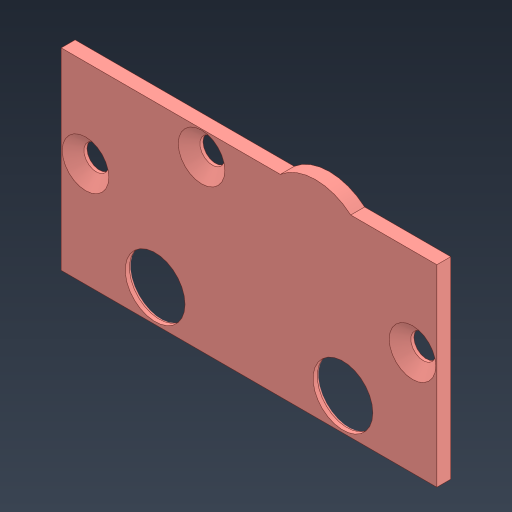
# Autodesk Inventor part: gearbox-wall-left
Saved by Autodesk Inventor 2023 (Build 270158000, 158)
## iProperties
Created: 2025-04-19
Part Number: gearbox-wall-left
Material: Generic
Document SubType Name: Modeling
Designer: szymo
Density: 1 g/cm^3
Appearance: Default(1)
Mass: 2.53528 g
Surface Area: 31.5747 cm^2
Volume: 2.53528 cm^3
Author: szymo
Autodesk Inventor part; units mm, degrees
ref_plane "YZ Plane" through (0, 0, 0) normal (1, 0, 0) x (0, 1, 0)
ref_plane "XZ Plane" through (0, 0, 0) normal (0, 1, 0) x (-1, 0, 0)
ref_plane "XY Plane" through (0, 0, 0) normal (0, 0, 1) x (1, 0, 0)
sketch "Sketch1" plane through (0, 0, 0) normal (0, 0, 1) x (1, 0, 0)
  circle A0 centre (-23.5, 0.7602) radius 2.5 projected
  circle A1 centre (23.5, 0.7602) radius 2.5 projected
  circle A2 centre (-6.8229, 9.9421) radius 2.5 projected
  arc A3 (-6.2914, -1.4253) -> (-23.3552, -14.2579) centre (-13.5, -9.6013) ccw projected
  arc A4 (-4.408, 0.1593) -> (-6.2914, -1.4253) centre (0, -6.9912) ccw projected
  arc A5 (23.3552, -14.2579) -> (18.5289, 0.0693) centre (13.5, -9.6013) ccw projected
  line L0 (-27, -14.2579) -> (27, -14.2579)
  circle A6 centre (-13.5, -9.6013) radius 6 projected
  circle A7 centre (13.5, -9.6013) radius 6 projected
  circle A8 centre (-13.5, -9.6013) radius 6.3
  circle A9 centre (13.5, -9.6013) radius 6.3
  arc A10 (15.8884, 4.2462) -> (2.7919, 9.881) centre (9.5585, 7.571) ccw projected
  arc A11 (18.5289, 0.0693) -> (15.8884, 4.2462) centre (13.15, -0.4079) ccw projected
  line L1 (23.3552, -14.2579) -> (27, -14.2579) projected
  line L2 (27, -14.2579) -> (27, 13.4421) projected
  line L3 (27, 13.4421) -> (14.6174, 13.4421) projected
  arc A12 (14.6174, 13.4421) -> (4.4995, 13.4421) centre (9.5585, 7.571) ccw projected
  line L4 (4.4995, 13.4421) -> (-27, 13.4421) projected
  line L5 (-27, 13.4421) -> (-27, -14.2579) projected
  line L6 (-27, -14.2579) -> (-23.3552, -14.2579) projected
  arc A13 (2.7919, 9.881) -> (-4.408, 0.1593) centre (2.2557, 2.7511) ccw projected
  point P0 (0, 0)
  point P1 (4.2365, 13.4421)
  point P2 (-17.7433, -14.2579)
  point P3 (-9.2567, -14.2579)
  point P4 (9.2567, -14.2579)
  point P5 (17.7433, -14.2579)
  point P6 (-23.3552, -14.2579)
  point P7 (23.3552, -14.2579)
  dimension "d0" = 0.3
  dimension "d1" = 0.3
  constraints: 2 centre point, 2 end point
  measures "d0" radial gap between concentric circles of A6 A8
  measures "d1" radial gap between concentric circles of A7 A9
ref_plane "Work Plane1" through (-19.5, -15.6013, 1) normal (0, 0, 1) x (1, 0, 0)
extrude "Extrusion1" add sketch "Sketch1" along normal up to surface (1 mm away) contours A0 | A1 | A2 | A4 A13 A10 A11 A5 L0 A9 A8 A3 | A3 L0 L5 L4 A12 L3 L2 A5 A11 A10 A13 A4
sketch "Sketch2" plane through (-27, 13.4421, 1) normal (0, 0, 1) x (1, 0, 0)
  line L0 (36.2567, -27.7) -> (17.7433, -27.7) projected
  circle A0 centre (13.5, -23.0433) radius 4 projected
  circle A1 centre (40.5, -23.0433) radius 4 projected
  arc A2 (17.7433, -27.7) -> (9.2567, -27.7) centre (13.5, -23.0433) ccw projected
  line L1 (9.2567, -27.7) -> (17.7433, -27.7)
  line L2 (36.2567, -27.7) -> (44.7433, -27.7)
  arc A3 (44.7433, -27.7) -> (36.2567, -27.7) centre (40.5, -23.0433) ccw projected
  circle A4 centre (13.5, -23.0433) radius 4.3
  circle A5 centre (40.5, -23.0433) radius 4.3
  line L3 (9.2567, -27.7) -> (0, -27.7) projected
  arc A6 (17.7433, -27.7) -> (9.2567, -27.7) centre (13.5, -23.0433) ccw projected
  arc A7 (44.7433, -27.7) -> (36.2567, -27.7) centre (40.5, -23.0433) ccw projected
  line L4 (54, -27.7) -> (44.7433, -27.7) projected
  line L5 (54, 0) -> (54, -27.7) projected
  line L6 (41.6174, 0) -> (54, 0) projected
  arc A8 (41.6174, 0) -> (31.4995, 0) centre (36.5585, -5.8711) ccw projected
  line L7 (0, 0) -> (31.4995, 0) projected
  line L8 (0, -27.7) -> (0, 0) projected
  point P0 (27, -13.4421)
  dimension "d4" = 0.3
  dimension "d5" = 0.3
  constraints: 4 end point, 2 centre point, 1 collinear, 1 point on circle
  measures "d4" radial gap between concentric circles of A0 A4
  measures "d5" radial gap between concentric circles of A1 A5
ref_plane "Work Plane2" through (-17.5, -13.6013, 2) normal (0, 0, 1) x (1, 0, 0)
extrude "Extrusion2" add sketch "Sketch2" along normal up to surface (1 mm away) contours A3 L2 | L0 A2 L3 L8 L7 A8 L6 L5 L4 A3 | L1 A2
sketch "Sketch3" plane through (-27, -14.2579, 2) normal (0, 0, 1) x (1, 0, 0)
  circle A0 centre (3.5, 15.0181) radius 2.5 projected
  circle A1 centre (50.5, 15.0181) radius 2.5 projected
  circle A2 centre (20.1771, 24.2) radius 2.5 projected
  arc A3 (20.7086, 12.8326) -> (3.6448, 0) centre (13.5, 4.6567) ccw projected
  arc A4 (22.592, 14.4172) -> (20.7086, 12.8326) centre (27, 7.2667) ccw projected
  arc A5 (50.3552, 0) -> (45.5289, 14.3273) centre (40.5, 4.6567) ccw projected
  arc A6 (42.8884, 18.5041) -> (29.7919, 24.1389) centre (36.5585, 21.8289) ccw projected
  arc A7 (45.5289, 14.3273) -> (42.8884, 18.5041) centre (40.15, 13.85) ccw projected
  line L0 (50.3552, 0) -> (54, 0) projected
  line L1 (54, 0) -> (54, 27.7) projected
  line L2 (54, 27.7) -> (41.6174, 27.7) projected
  arc A8 (41.6174, 27.7) -> (31.4995, 27.7) centre (36.5585, 21.8289) ccw projected
  line L3 (31.4995, 27.7) -> (0, 27.7) projected
  line L4 (0, 27.7) -> (0, 0) projected
  line L5 (0, 0) -> (3.6448, 0) projected
  arc A9 (29.7919, 24.1389) -> (22.592, 14.4172) centre (29.2557, 17.009) ccw projected
  point P0 (27, 14.2579)
  point P1 (31.2365, 27.7)
  point P2 (3.5, 15.0181)
  point P3 (20.1771, 24.2)
  point P4 (50.5, 15.0181)
  constraints: 3 coincident
hole "Hole1" at (-23.5, 0.7602, 2) at (-6.8229, 9.9421, 2) at (23.5, 0.7602, 2) direction (0, 0, -1) diameter 3.6 depth 4 countersink diameter 6.7 countersink angle 90 clearance for "Countersunk Flat Head Screw ISO 2009/7046" size "M3" standard "ISO"
fillet "Fillet1" radius 0.4 4 edges at (9.2, -9.6013, 1) (13.5, -3.3013, 0) (-17.8, -9.6013, 1) (-13.5, -3.3013, 0)
sketch "Sketch4" plane through (0, 0, 0) normal (0, 0, -1) x (-1, 0, 0)
  circle A0 centre (0, -6.9912) radius 1.25 projected
  circle A1 centre (-2.2557, 2.7511) radius 1.25 projected
  circle A2 centre (-9.5585, 7.571) radius 1.25 projected
  circle A3 centre (-9.5585, 7.571) radius 1.45
  circle A4 centre (-2.2557, 2.7511) radius 1.45
  circle A5 centre (0, -6.9912) radius 1.45
  point P0 (0, 0)
  dimension "d16" = 0.2
  dimension "d17" = 0.2
  dimension "d18" = 0.2
  constraints: 3 centre point
  measures "d16" radial gap between concentric circles of A2 A3
  measures "d17" radial gap between concentric circles of A1 A4
  measures "d18" radial gap between concentric circles of A0 A5
extrude "Extrusion3" cut sketch "Sketch4" against normal blind 1.4 contours A0 | A1 | A2 | A3 | A4 | A5
fillet "Fillet2" radius 0.4 3 edges at (1.45, -6.9912, 0) (3.7057, 2.7511, 0) (11.0085, 7.571, 0)
body "Solid1"
